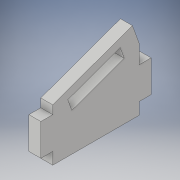
# Autodesk Inventor part: k_thumb_profile
Saved by Autodesk Inventor 2017 (Build 210142000, 142)
## iProperties
Created: 2017-02-08
Part Number: k_thumb_profile
Material: Generic
Document SubType Name: Modeling
Designer: herman
Density: 1 g/cm^3
Appearance: Default
Author: herman
Autodesk Inventor part; units mm, degrees
ref_plane "YZ Plane" through (0, 0, 0) normal (1, 0, 0) x (0, 1, 0)
ref_plane "XZ Plane" through (0, 0, 0) normal (0, 1, 0) x (-1, 0, 0)
ref_plane "XY Plane" through (0, 0, 0) normal (0, 0, 1) x (1, 0, 0)
sketch "Sketch2" plane through (0, 0, 0) normal (1, 0, 0) x (0, 1, 0)
  line L0 (16.0342, 2.2983) -> (13.213, 1.278)
  line L1 (13.213, 1.278) -> (17.9745, -11.8874)
  line L2 (17.9745, -11.8874) -> (20.7956, -10.8671)
  line L3 (20.7956, -10.8671) -> (16.0342, 2.2983)
  line L4 (16.8006, 6.0599) -> (24.0368, -13.9485)
  line L5 (14.6738, 6.0599) -> (16.8006, 6.0599)
  line L6 (24.0368, -13.9485) -> (19.3349, -15.649)
  line L7 (19.3349, -15.649) -> (14.6738, -15.649)
  line L8 (22.156, -14.6287) -> (14.6738, 6.0599) construction
  line L9 (17.9745, -11.8874) -> (11.3917, -14.2681) construction
  line L10 (11.3917, -14.2681) -> (6.6303, -1.1027) construction
  line L11 (6.6303, -1.1027) -> (13.213, 1.278) construction
  line L12 (6.6738, 6.0599) -> (3.6738, 6.0599)
  line L13 (3.6738, 6.0599) -> (3.6738, -15.649)
  line L14 (3.6738, -15.649) -> (6.6738, -15.649)
  line L15 (14.6738, 6.0599) -> (14.6738, 9.0599)
  line L16 (14.6738, 9.0599) -> (6.6738, 9.0599)
  line L17 (6.6738, 9.0599) -> (6.6738, 6.0599)
  line L18 (6.6738, -15.649) -> (6.6738, -18.649)
  line L19 (6.6738, -18.649) -> (14.6738, -18.649)
  line L20 (14.6738, -18.649) -> (14.6738, -15.649)
  point P0 (0, 0)
  dimension "d9" = 5
  dimension "d11" = 2
  dimension "d13" = 4
  dimension "d14" = 4
  dimension "d15" = 14
  dimension "d16" = 7
  dimension "d17" = 3
  dimension "d18" = 3
  dimension "d21" = 3
  dimension "d22" = 3
  dimension "d27" = 21.7089
  dimension "d28" = 8
  dimension "d29" = 8
  constraints: 42 end point, 12 perpendicular, 6 parallel, 3 horizontal, 3 point on line, 1 vertical
  measures "d9" distance of L4.end L6.end
  measures "d11" distance between parallel lines of L4 L3
  measures "d13" distance between parallel lines of L6 L2
  measures "d14" distance of L5.start L0.start
  measures "d15" distance of L2.end L0.start
  measures "d16" distance of L1.end L9.end
  measures "d17" distance of L13.end L14.end
  measures "d18" distance between parallel lines of L1 L3
  measures "d21" distance of L19.end L7.end
  measures "d22" distance of L5.start L15.end
  measures "d27" distance of L13.end L12.end
  measures "d28" distance of L15.end L16.end
  measures "d29" distance of L18.end L19.end
extrude "Extrusion1" add sketch "Sketch2" along normal blind 3
equation "\"d13\" = d14"
body "Solid2"
